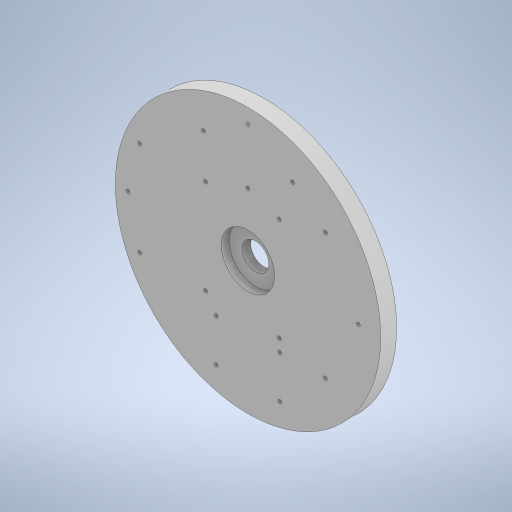
# Autodesk Inventor part: base_board
Saved by Autodesk Inventor 2023 (Build 270158000, 158)
## iProperties
Created: 2023-05-20
Part Number: base_board
Material: 一般
Document SubType Name: Modeling
Designer: 310611102
Density: 1 g/cm^3
Appearance: 預設
Author: 310611102
Autodesk Inventor part; units mm, degrees
ref_plane "YZ Plane" through (0, 0, 0) normal (1, 0, 0) x (0, 1, 0)
ref_plane "XZ Plane" through (0, 0, 0) normal (0, 1, 0) x (-1, 0, 0)
ref_plane "XY Plane" through (0, 0, 0) normal (0, 0, 1) x (1, 0, 0)
sketch "Sketch1" plane through (0, 0, 0) normal (0, 0, 1) x (1, 0, 0)
  circle A0 centre (0, 0) radius 125
  dimension "d0" = 250
  constraints: 1 centre point, 1 coincident
  measures "d0" diameter of A0
extrude "Extrusion1" add sketch "Sketch1" along normal blind 15
sketch "Sketch2" plane through (0, 0, 15) normal (0, 0, 1) x (1, 0, 0)
  circle A0 centre (0, 0) radius 25
  dimension "d3" = 50
  constraints: 1 centre point, 1 coincident
  measures "d3" diameter of A0
extrude "Extrusion2" cut sketch "Sketch2" against normal blind 7
sketch "Sketch3" plane through (0, 0, 8) normal (0, 0, 1) x (1, 0, 0)
  circle A0 centre (0, 0) radius 12.5
  dimension "d6" = 25
  constraints: 1 centre point, 1 coincident
  measures "d6" diameter of A0
extrude "Extrusion3" cut sketch "Sketch3" against normal through all
sketch "Sketch4" plane through (0, 0, 15) normal (0, 0, 1) x (1, 0, 0)
  circle A0 centre (29.5, -48.5) radius 1.6
  line L0 (0, 0) -> (147.2327, 0)
  line L1 (73, 0) -> (73, 59.5)
  circle A1 centre (29.5, 48.5) radius 1.6
  circle A2 centre (73, -59.5) radius 1.6
  circle A3 centre (73, 59.5) radius 1.6
  circle A4 centre (104, 0) radius 1.6
  dimension "d11" = 3.2
  dimension "d50" = 73
  dimension "d51" = 3.2
  dimension "d52" = 43.5
  dimension "d53" = 3.2
  dimension "d54" = 31
  dimension "d55" = 97
  dimension "d56" = 119
  constraints: 5 centre point, 4 end point, 2 point on line, 2 symmetric about line, 1 coincident, 1 horizontal, 1 vertical, 2 other
  measures "d11" diameter of A0
  measures "d50" horizontal distance of L1.end L0.start
  measures "d51" diameter of A2
  measures "d52" horizontal distance of L1.start A0.centre
  measures "d53" diameter of A4
  measures "d54" distance of A4.centre L1.start
  measures "d55" distance of A1.centre A0.centre
  measures "d56" distance of A3.centre A2.centre
extrude "Extrusion4" cut sketch "Sketch4" against normal blind 8
sketch "Sketch5" plane through (0, 0, 15) normal (0, 0, 1) x (1, 0, 0)
  line L0 (-43.6176, 0) -> (7.6417, 0)
  circle A0 centre (-40, 44.5) radius 1.6
  circle A1 centre (-40, -44.5) radius 1.6
  line L1 (-71, 46.1) -> (-71, -32.5719)
  circle A2 centre (-102, 44.5) radius 1.6
  circle A3 centre (-102, -44.5) radius 1.6
  circle A4 centre (-113, 0) radius 1.6
  point P0 (0, 0)
  dimension "d60" = 3.2
  dimension "d61" = 89
  dimension "d62" = 62
  dimension "d63" = 40
  dimension "d64" = 3.2
  dimension "d65" = 11
  constraints: 5 centre point, 4 end point, 3 symmetric about line, 1 horizontal, 1 horizontal alignment, 1 point on line, 1 vertical, 3 other
  measures "d60" diameter of A0
  measures "d61" distance of A1.centre A0.centre
  measures "d62" distance of A0.centre A2.centre
  measures "d63" horizontal distance of point (0, 0) A0.centre
  measures "d64" diameter of A4
  measures "d65" horizontal distance of A2.centre A4.centre
extrude "Extrusion5" cut sketch "Sketch5" against normal blind 8
sketch "Sketch6" plane through (0, 0, 15) normal (0, 0, 1) x (1, 0, 0)
  circle A0 centre (-42, 85) radius 1.6
  line L0 (0, 131.4928) -> (0, 57.1829)
  line L1 (-43.3756, 85) -> (37.4091, 85)
  circle A1 centre (42, 85) radius 1.6
  circle A2 centre (0, 111) radius 1.6
  circle A3 centre (0, 59) radius 1.6
  point P0 (0, 0)
  dimension "d38" = 3.2
  dimension "d85" = 85
  dimension "d86" = 84
  dimension "d87" = 3.2
  dimension "d88" = 52
  constraints: 4 centre point, 4 end point, 3 point on line, 2 symmetric about line, 1 horizontal, 1 vertical, 2 other
  measures "d38" diameter of A0
  measures "d85" vertical distance of point (0, 0) L1.end
  measures "d86" distance of A1.centre A0.centre
  measures "d87" diameter of A2
  measures "d88" distance of A3.centre A2.centre
extrude "Extrusion6" cut sketch "Sketch6" against normal blind 8
sketch "Sketch9" plane through (0, 0, 15) normal (0, 0, 1) x (1, 0, 0)
  line L0 (0, -68.2489) -> (0, -119.1894)
  line L1 (-34.7906, -80) -> (35.8893, -80)
  circle A0 centre (-30, -60) radius 1.6
  circle A1 centre (30, -60) radius 1.6
  circle A2 centre (-30, -100) radius 1.6
  circle A3 centre (30, -100) radius 1.6
  point P0 (0, 0)
  point P1 (0.5493, -80)
  dimension "d77" = 80
  dimension "d78" = 3.2
  dimension "d79" = 60
  dimension "d89" = 40
  constraints: 4 centre point, 4 end point, 3 symmetric about line, 1 horizontal, 1 midpoint, 1 point on line, 1 vertical, 3 other
  measures "d77" vertical distance of L1.start point (0, 0)
  measures "d78" diameter of A0
  measures "d79" diameter of A0.centre L0
  measures "d89" distance of A2.centre A0.centre
extrude "Extrusion8" cut sketch "Sketch9" against normal blind 8
sketch "Sketch7" plane through (0, 0, 0) normal (0, 0, -1) x (-1, 0, 0)
  circle A0 centre (77.5, 42.5) radius 1.6
  circle A1 centre (0, 0) radius 12.5 projected
  line L0 (0, 0) -> (77.5, 0)
  circle A2 centre (77.5, -42.5) radius 1.6
  line L1 (0, 0) -> (26.3155, 0)
  line L2 (77.5, 42.5) -> (77.5, -42.5)
  dimension "d66" = 3.2
  dimension "d67" = 85
  dimension "d75" = 0
  dimension "d76" = 77.5
  constraints: 6 end point, 2 centre point, 2 coincident, 1 horizontal, 1 midpoint, 1 perpendicular, 1 symmetric about line, 1 other
  measures "d66" diameter of A0
  measures "d67" distance of A2.centre A0.centre
  measures "d75" distance between parallel lines of L1 L0
  measures "d76" distance of L0.end L0.start
extrude "Extrusion7" cut sketch "Sketch7" against normal blind 8 contours A0 | A2
pattern_circular "Circular Pattern1" count 4 over 360 about axis through (0, 0, 8) along (0, 0, -1) of "Extrusion7"
sketch "Sketch8" plane through (0, 0, 15) normal (0, 0, 1) x (1, 0, 0)
  point P0 (0, 0)
body "Solid1"
